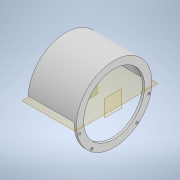
# Autodesk Inventor part: Крышка на мотор
Saved by Autodesk Inventor 2022.1 (Build 261234000, 234)
## iProperties
Created: 2021-12-25
Part Number: Крышка на мотор
Material: Типовые
Document SubType Name: Modeling
Designer: Grigori
Density: 1 g/cm^3
Appearance: По умолчанию
Author: Grigori
Autodesk Inventor part; units mm, degrees
ref_plane "YZ Plane" through (0, 0, 0) normal (1, 0, 0) x (0, 1, 0)
ref_plane "XZ Plane" through (0, 0, 0) normal (0, 1, 0) x (-1, 0, 0)
ref_plane "XY Plane" through (0, 0, 0) normal (0, 0, 1) x (1, 0, 0)
sketch "Эскиз1" plane through (0, 0, 0) normal (1, 0, 0) x (0, 1, 0)
  circle A0 centre (37.5, 47.7) radius 39.7
  circle A1 centre (37.5, 47.7) radius 39.7
  circle A2 centre (37.5, 47.7) radius 49.1718
  point P0 (0, 0)
  constraints: 3 centre point, 2 coincident, 1 concentric
extrude "Выдавливание1" add sketch "Эскиз1" along normal blind 3
sketch "Эскиз2" plane through (0, 37.5, 47.7) normal (-1, 0, 0) x (0, 0, 1)
  arc A0 (42.2878, 5.9187) -> (-42.2878, 5.9187) centre (0, 0) ccw
  arc A1 (-42.2878, 5.9187) -> (-49.1127, 2.4088) centre (0, -84.7) ccw
  arc A2 (49.1127, 2.4088) -> (42.2878, 5.9187) centre (0, -84.7) ccw
  arc A3 (49.1127, 2.4088) -> (-49.1127, 2.4088) centre (0, 0) ccw
  constraints: 8 point on circle, 4 centre point, 1 coincident
extrude "Выдавливание2" add sketch "Эскиз2" along normal blind 60
sketch "Эскиз3" plane through (3, 37.5, 47.7) normal (1, 0, 0) x (0, 0, -1)
  circle A0 centre (0, 0) radius 39.7 projected
  circle A1 centre (-45.186, -10.976) radius 1.5
  circle A2 centre (-29.3932, -36.0318) radius 1.5
  circle A3 centre (45.186, -10.976) radius 1.5
  circle A4 centre (29.3932, -36.0318) radius 1.5
  point P0 (47.7, -37.5)
  dimension "d9" = 3
  dimension "d10" = 3
  constraints: 4 centre point
  measures "d9" diameter of A1
  measures "d10" diameter of A2
extrude "Выдавливание4" cut sketch "Эскиз3" against normal blind 60 contours A1 | A2 | A3 | A4
sketch "Эскиз4" plane through (-60, 37.5, 47.7) normal (-1, 0, 0) x (0, 0, 1)
  arc A0 (-42.2878, 5.9187) -> (-49.1127, 2.4088) centre (0, -84.7) ccw projected
  arc A1 (42.2878, 5.9187) -> (-42.2878, 5.9187) centre (0, -84.7) ccw
  arc A2 (42.1214, 7.1077) -> (-42.1214, 7.1077) centre (0, -84.7) ccw
  line L0 (0, 16.3092) -> (0.5, 16.308)
  line L1 (0.5, 16.308) -> (-0.5, 16.3092)
  arc A3 (42.2878, 5.9187) -> (-42.2878, 5.9187) centre (0, 0) ccw projected
  line L2 (42.1214, 7.1077) -> (42.2878, 5.9187)
  line L3 (-42.1214, 7.1077) -> (-42.2878, 5.9187)
  point P0 (-47.7, -37.5)
  point P1 (-0.25, 16.3089)
  dimension "d14" = 0.5
  dimension "d15" = 1
  constraints: 8 end point, 6 point on circle, 2 centre point, 2 coincident, 3 other
  measures "d14" distance of L0.start L0.end
  measures "d15" distance of L0.end L1.end
extrude "Выдавливание5" add sketch "Эскиз4" against normal blind 2 contours A1 A3 A2 | A3 A2 L2 | L3 A2 A3
sketch "Эскиз6" plane through (-60, 37.5, 47.7) normal (-1, 0, 0) x (0, 0, 1)
  arc A0 (42.1029, 7.1162) -> (-42.1029, 7.1162) centre (0, 0) ccw projected
  arc A1 (42.1029, 7.1162) -> (-42.1029, 7.1162) centre (0, -84.7) ccw projected
  line L0 (0, 16.3092) -> (-0.5, 16.3092)
  line L1 (0, 16.3092) -> (0.5, 16.3092) construction
  line L2 (-0.5, 16.3092) -> (0.5, 16.3092)
  line L3 (0.5, 16.3092) -> (0.5, 42.6971)
  line L4 (0.5, 42.6971) -> (-0.5, 42.6971)
  line L5 (0.5, 42.6971) -> (1.5, 42.6971) construction
  line L6 (-0.5, 42.6971) -> (-0.5, 16.3092)
  point P0 (-47.7, -37.5)
  dimension "d25" = 0.5
  dimension "d26" = 180
  dimension "d27" = 1
  dimension "d28" = 0
  dimension "d29" = 1
  dimension "d30" = 180
  constraints: 14 end point, 4 horizontal, 3 collinear, 2 point on circle, 1 perpendicular, 1 tangent
  measures "d25" distance of L0.start L0.end
  measures "d26" angle of L0 L1
  measures "d27" distance of L0.end L2.end
  measures "d28" distance between parallel lines of L2 L0
  measures "d29" distance of L3.end L4.end
  measures "d30" angle of L4 L5
extrude "Выдавливание7" add sketch "Эскиз6" against normal blind 2 contours L3 A1 L6 L4
pattern_circular "Круговой массив1" count 300 over 360 about axis through (-60, -47.2, 47.7) along (1, 0, 0) of "Выдавливание7"
sketch "Эскиз7" plane through (-60, 37.5, 47.7) normal (-1, 0, 0) x (0, 0, 1)
  circle A0 centre (0, 0) radius 237.0324
  arc A1 (-49.1127, 2.4088) -> (49.1127, 2.4088) centre (0, 0) ccw projected
  circle A2 centre (0, 0) radius 49.1718
  point P0 (-47.7, -37.5)
  point P1 (-49.1127, 2.4088)
  point P2 (49.1127, 2.4088)
  constraints: 2 centre point, 1 coincident, 1 concentric
extrude "Выдавливание8" cut sketch "Эскиз7" along normal through all both and the other way through all
ref_plane "РабПлоскость6" through (1.5, 37.5, 47.7) normal (1, 0, 0) x (0, 0, -1)
ref_plane "РабПлоскость7" through (-30, 37.5, 47.7) normal (-1, 0, 0) x (0, 0, 1)
ref_plane "РабПлоскость5" through (1.5, 35.0974, 62.4739) normal (0, 1, 0) x (0, 0, -1)
sketch "Эскиз10" plane through (1.5, 35.0974, 62.4739) normal (0, 1, 0) x (0, 0, -1)
  line L0 (-34.3978, 1.5) -> (63.9457, 1.5) projected
  line L1 (14.7739, 1.5) -> (14.7739, 83.7421)
  line L2 (14.7739, 1.5) -> (-31.1261, 1.5)
  circle A0 centre (-31.1261, 51.234) radius 1.5
  circle A1 centre (-31.1261, 32.434) radius 1.5
  circle A2 centre (-31.1261, 14.694) radius 1.5
  circle A3 centre (60.6739, 51.234) radius 1.5
  circle A4 centre (60.6739, 32.434) radius 1.5
  circle A5 centre (60.6739, 14.694) radius 1.5
  point P0 (62.4739, 1.5)
  point P1 (-34.3388, 1.5)
  point P2 (63.8866, 1.5)
  dimension "d39" = 45.9
  dimension "d43" = 3
  dimension "d44" = 3
  dimension "d45" = 3
  constraints: 6 centre point, 4 end point, 3 symmetric about line, 1 midpoint, 1 point on line, 1 vertical, 3 other
  measures "d39" distance of L1.start L2.end
  measures "d43" diameter of A0
  measures "d44" diameter of A1
  measures "d45" diameter of A2
extrude "Выдавливание9" cut sketch "Эскиз10" along normal blind 10
thread "Резьба1" size "M3x0.5" class "6H" standard "ANSI Metric M Profile" full length
thread "Резьба2" size "M3x0.5" class "6H" standard "ANSI Metric M Profile" full length
thread "Резьба3" size "M3x0.5" class "6H" standard "ANSI Metric M Profile" full length
thread "Резьба4" size "M3x0.5" class "6H" standard "ANSI Metric M Profile" full length
thread "Резьба5" size "M3x0.5" class "6H" standard "ANSI Metric M Profile" full length
thread "Резьба6" size "M3x0.5" class "6H" standard "ANSI Metric M Profile" full length
